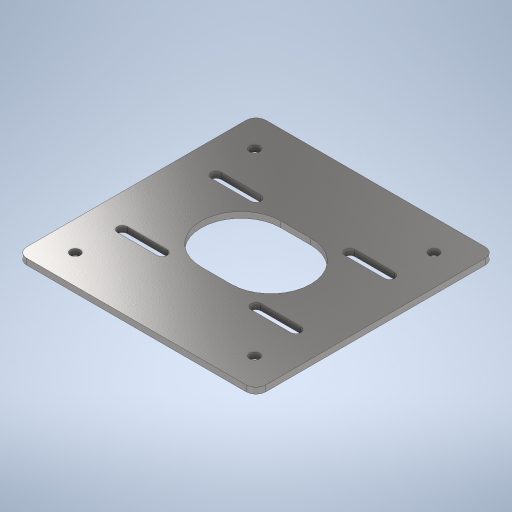
# Autodesk Inventor part: motormountplate
Saved by Autodesk Inventor 2024 (Build 280153000, 153)
## iProperties
Created: 2023-12-19
Part Number: motormountplate
Material: Steel, Galvanized
Document SubType Name: Modeling
Designer: weiti
Density: 7.85 g/cm^3
Appearance: Galvanized
Author: weiti
Autodesk Inventor part; units mm, degrees
ref_plane "YZ Plane" through (0, 0, 0) normal (1, 0, 0) x (0, 1, 0)
ref_plane "XZ Plane" through (0, 0, 0) normal (0, 1, 0) x (-1, 0, 0)
ref_plane "XY Plane" through (0, 0, 0) normal (0, 0, 1) x (1, 0, 0)
sketch "Sketch1" plane through (0, 0, 0) normal (0, 1, 0) x (-1, 0, 0)
  line L0 (60, 60) -> (-60, 60)
  line L1 (-60, 60) -> (-60, -60)
  line L2 (-60, -60) -> (60, -60)
  line L3 (60, -60) -> (60, 60)
  line L4 (60, 60) -> (-60, -60) construction
  line L5 (-60, 60) -> (60, -60) construction
  line L6 (60, 0) -> (-60, 0)
  line L7 (0, 60) -> (0, -60)
  circle A0 centre (45.3511, 45.3511) radius 2.5
  circle A1 centre (45.3511, -44.6489) radius 2.5
  circle A2 centre (-44.6489, 45.3511) radius 2.5
  circle A3 centre (-44.6489, -44.6489) radius 2.5
  line L8 (7.5, 0) -> (-7.5, 0) construction
  line L9 (7.5, 20) -> (-7.5, 20)
  line L10 (-7.5, -20) -> (7.5, -20)
  arc A4 (7.5, -20) -> (7.5, 20) centre (7.5, 0) ccw
  arc A5 (-7.5, 20) -> (-7.5, -20) centre (-7.5, 0) ccw
  line L11 (43.55, 23.55) -> (23.55, 23.55) construction
  line L12 (43.55, 26.05) -> (23.55, 26.05)
  line L13 (23.55, 21.05) -> (43.55, 21.05)
  arc A6 (43.55, 21.05) -> (43.55, 26.05) centre (43.55, 23.55) ccw
  arc A7 (23.55, 26.05) -> (23.55, 21.05) centre (23.55, 23.55) ccw
  line L14 (43.55, -23.55) -> (23.55, -23.55) construction
  line L15 (43.55, -26.05) -> (23.55, -26.05)
  line L16 (23.55, -21.05) -> (43.55, -21.05)
  arc A8 (43.55, -26.05) -> (43.55, -21.05) centre (43.55, -23.55) ccw
  arc A9 (23.55, -21.05) -> (23.55, -26.05) centre (23.55, -23.55) ccw
  line L17 (-43.55, 23.55) -> (-23.55, 23.55) construction
  line L18 (-43.55, 26.05) -> (-23.55, 26.05)
  line L19 (-23.55, 21.05) -> (-43.55, 21.05)
  arc A10 (-43.55, 26.05) -> (-43.55, 21.05) centre (-43.55, 23.55) ccw
  arc A11 (-23.55, 21.05) -> (-23.55, 26.05) centre (-23.55, 23.55) ccw
  line L20 (-23.55, -21.05) -> (-43.55, -21.05)
  line L21 (-43.55, -23.55) -> (-23.55, -23.55) construction
  arc A12 (-23.55, -26.05) -> (-23.55, -21.05) centre (-23.55, -23.55) ccw
  arc A13 (-43.55, -21.05) -> (-43.55, -26.05) centre (-43.55, -23.55) ccw
  line L22 (-43.55, -26.05) -> (-23.55, -26.05)
  point P0 (0, 0)
  point P1 (0, 0)
  point P2 (33.55, 23.55)
  point P3 (33.55, -23.55)
  point P4 (33.55, -23.55)
  point P5 (-33.55, 23.55)
  point P6 (-33.55, -23.55)
  point P7 (-33.55, -23.55)
  dimension "d2" = 120
  dimension "d3" = 120
  dimension "d4" = 5
  dimension "d7" = 90
  dimension "d10" = 90
  dimension "d13" = 15
  dimension "d14" = 7.5
  dimension "d15" = 20
  dimension "d16" = 20
  dimension "d17" = 2.5
  dimension "d18" = 47.1
  constraints: 56 end point, 22 symmetric about line, 20 point on circle, 14 centre point, 9 midpoint, 8 tangent, 4 parallel, 4 point on line, 3 horizontal, 1 perpendicular, 1 vertical, 12 other
  measures "d2" distance of L2.end L1.end
  measures "d3" distance of L2.end L0.start
  measures "d4" diameter of A0
  measures "d7" distance of A0.centre A1.centre
  measures "d10" distance of A0.centre A2.centre
  measures "d13" distance of L9.start L9.end
  measures "d14" distance from line of L7 L8.start
  measures "d15" radius of A5
  measures "d16" distance of L12.start L12.end
  measures "d17" radius of A6
  measures "d18" distance of point (33.55, -23.55) point (33.55, 23.55)
extrude "Extrusion1" add sketch "Sketch1" along normal blind 3 contours L3 L6 A4 L9 L7 L0 | L7 L9 A5 L6 L1 L0 | L3 L2 L7 L10 A4 L6 | L6 A5 L10 L7 L2 L1
fillet "Fillet1" radius 5 4 edges at (60, 1.5, -60) (-60, 1.5, -60) (-60, 1.5, 60) (60, 1.5, 60)
body "Solid1"
